Autodesk Fusion 360 part; units mm, degrees
(part 2 of 3)
sketch "Sketch4" plane through (0, 0, 0) normal (0, -1, 0) x (1, 0, 0)
  circle A0 centre (0, 8) radius 4.5
  circle A1 centre (0, 35) radius 5.25
  line L0 (-36.5, 36.5) -> (-36.5, -36.5)
  line L1 (-36.5, -36.5) -> (36.5, -36.5)
  line L2 (36.5, -36.5) -> (36.5, 36.5)
  arc A2 (36.5, 36.5) -> (-36.5, 36.5) centre (0, 36.5) ccw
  line L3 (35, -35) -> (28.75, -35)
  line L4 (28.75, -35) -> (28.75, -30)
  line L5 (28.75, -30) -> (35, -30)
  line L6 (35, -30) -> (35, -35)
  line L7 (28.75, -30) -> (13.75, -30)
  line L8 (13.75, -30) -> (13.75, -20)
  line L9 (13.75, -20) -> (28.75, -20)
  line L10 (28.75, -20) -> (28.75, -30)
  line L11 (13.75, -30) -> (7.5, -30)
  line L12 (7.5, -30) -> (7.5, -35)
  line L13 (7.5, -35) -> (13.75, -35)
  line L14 (13.75, -35) -> (13.75, -30)
  line L15 (7.5, -30) -> (-7.5, -30)
  line L16 (-7.5, -30) -> (-7.5, -20)
  line L17 (-7.5, -20) -> (7.5, -20)
  line L18 (7.5, -20) -> (7.5, -30)
  line L19 (-7.5, -30) -> (-13.75, -30)
  line L20 (-13.75, -30) -> (-13.75, -35)
  line L21 (-13.75, -35) -> (-7.5, -35)
  line L22 (-7.5, -35) -> (-7.5, -30)
  line L23 (-13.75, -30) -> (-28.75, -30)
  line L24 (-28.75, -30) -> (-28.75, -20)
  line L25 (-28.75, -20) -> (-13.75, -20)
  line L26 (-13.75, -20) -> (-13.75, -30)
  line L27 (-28.75, -30) -> (-35, -30)
  line L28 (-35, -30) -> (-35, -35)
  line L29 (-35, -35) -> (-28.75, -35)
  line L30 (-28.75, -35) -> (-28.75, -30)
  line L31 (28.75, -20) -> (35, -20)
  line L32 (35, -20) -> (35, -13.75)
  line L33 (35, -13.75) -> (28.75, -13.75)
  line L34 (28.75, -13.75) -> (28.75, -20)
  line L35 (28.75, -13.75) -> (13.75, -13.75)
  line L36 (13.75, -13.75) -> (13.75, -3.75)
  line L37 (13.75, -3.75) -> (28.75, -3.75)
  line L38 (28.75, -3.75) -> (28.75, -13.75)
  line L39 (13.75, -13.75) -> (7.5, -13.75)
  line L40 (7.5, -13.75) -> (7.5, -20)
  line L41 (7.5, -20) -> (13.75, -20)
  line L42 (13.75, -20) -> (13.75, -13.75)
  line L43 (7.5, -13.75) -> (-7.5, -13.75)
  line L44 (-7.5, -13.75) -> (-7.5, -3.75)
  line L45 (-7.5, -3.75) -> (7.5, -3.75)
  line L46 (7.5, -3.75) -> (7.5, -13.75)
  line L47 (-7.5, -13.75) -> (-13.75, -13.75)
  line L48 (-13.75, -13.75) -> (-13.75, -20)
  line L49 (-13.75, -20) -> (-7.5, -20)
  line L50 (-7.5, -20) -> (-7.5, -13.75)
  line L51 (-13.75, -13.75) -> (-28.75, -13.75)
  line L52 (-28.75, -13.75) -> (-28.75, -3.75)
  line L53 (-28.75, -3.75) -> (-13.75, -3.75)
  line L54 (-13.75, -3.75) -> (-13.75, -13.75)
  point P0 (35, -35)
  point P1 (-35, -35)
  dimension "d22" = 6.25
  dimension "d23" = 5
  dimension "d24" = 15
  dimension "d25" = 10
  dimension "d26" = 6.25
  dimension "d27" = 15
  dimension "d28" = 10
  dimension "d29" = 6.25
  dimension "d30" = 15
  dimension "d31" = 10
  dimension "d32" = 6.25
  dimension "d33" = 15
  dimension "d34" = 10
  dimension "d35" = 15
  dimension "d36" = 10
  dimension "d37" = 15
  dimension "d38" = 10
  constraint horizontal L3
  constraint vertical L4
  constraint horizontal L5
  constraint vertical L6
  constraint coincident P0 L3.start
  constraint horizontal L7
  constraint vertical L8
  constraint horizontal L9
  constraint vertical L10
  constraint horizontal L11
  constraint vertical L12
  constraint horizontal L13
  constraint vertical L14
  constraint horizontal L15
  constraint vertical L16
  constraint horizontal L17
  constraint vertical L18
  constraint horizontal L19
  constraint vertical L20
  constraint horizontal L21
  constraint vertical L22
  constraint horizontal L23
  constraint vertical L24
  constraint horizontal L25
  constraint vertical L26
  constraint horizontal L27
  constraint vertical L28
  constraint horizontal L29
  constraint vertical L30
  constraint coincident P1 L28.end
  constraint horizontal L31
  constraint vertical L32
  constraint horizontal L33
  constraint vertical L34
  constraint horizontal L35
  constraint vertical L36
  constraint horizontal L37
  constraint vertical L38
  constraint horizontal L39
  constraint vertical L40
  constraint horizontal L41
  constraint vertical L42
  constraint horizontal L43
  constraint vertical L44
  constraint horizontal L45
  constraint vertical L46
  constraint horizontal L47
  constraint vertical L48
  constraint horizontal L49
  constraint vertical L50
  constraint horizontal L51
  constraint vertical L52
  constraint horizontal L53
  constraint vertical L54
  measures "d22" distance of P0 L3.end
  measures "d23" distance of P0 L5.end
  measures "d24" distance of L4.end L7.end
  measures "d25" distance of L4.end L9.end
  measures "d26" distance of L7.end L11.end
  measures "d27" distance of L11.end L15.end
  measures "d28" distance of L11.end L17.end
  measures "d29" distance of L15.end L19.end
  measures "d30" distance of L19.end L23.end
  measures "d31" distance of L19.end L25.end
  measures "d32" distance of L9.end L33.end
  measures "d33" distance of L33.end L35.end
  measures "d34" distance of L33.end L37.end
  measures "d35" distance of L39.end L43.end
  measures "d36" distance of L39.end L45.end
  measures "d37" distance of L47.end L51.end
  measures "d38" distance of L47.end L53.end
extrude "Extrude6" cut sketch "Sketch4" against normal blind 3 contours L51 L52 L53 L54 | L7 L8 L9 L10 | L15 L16 L17 L18 | L35 L36 L37 L38 | L43 L44 L45 L46 | L23 L24 L25 L26 bodies 2
sketch "Sketch5" plane through (0, 0, -36.5) normal (0, 0, -1) x (-1, 0, 0)
  line L0 (36.5, 0) -> (-36.5, 0)
  line L1 (-36.5, 0) -> (-36.5, -25)
  line L2 (-36.5, -25) -> (36.5, -25)
  line L3 (36.5, -25) -> (36.5, 0)
  line L4 (36.5, -25) -> (24, -25)
  line L5 (24, -25) -> (24, -16)
  line L6 (24, -16) -> (36.5, -16)
  line L7 (36.5, -16) -> (36.5, -25)
  line L8 (24, -16) -> (11, -16)
  line L9 (11, -16) -> (11, -25)
  line L10 (11, -25) -> (24, -25)
  line L11 (24, -25) -> (24, -16)
  dimension "d41" = 12.5
  dimension "d42" = 9
  dimension "d43" = 13
  constraint horizontal L4
  constraint vertical L5
  constraint horizontal L6
  constraint vertical L7
  constraint coincident L2.end L3.start
  constraint horizontal L8
  constraint vertical L9
  constraint horizontal L10
  constraint vertical L11
  measures "d41" distance of L2.end L4.end
  measures "d42" distance of L2.end L6.end
  measures "d43" distance of L5.end L8.end
extrude "Extrude7" cut sketch "Sketch5" against normal blind 2 contours L2 L5 L8 L9 L10 L11 bodies 1
sketch "Sketch6" plane through (0, 0, 0) normal (0, -1, 0) x (1, 0, 0)
  line L0 (13.75, -13.75) -> (13.75, -3.75)
  line L1 (13.75, -3.75) -> (28.75, -3.75)
  line L2 (28.75, -3.75) -> (28.75, -13.75)
  line L3 (28.75, -13.75) -> (13.75, -13.75)
  line L4 (-28.75, -30) -> (-28.75, -20)
  line L5 (-28.75, -20) -> (-13.75, -20)
  line L6 (-13.75, -20) -> (-13.75, -30)
  line L7 (-13.75, -30) -> (-28.75, -30)
  line L8 (-7.5, -13.75) -> (-7.5, -3.75)
  line L9 (-7.5, -3.75) -> (7.5, -3.75)
  line L10 (7.5, -3.75) -> (7.5, -13.75)
  line L11 (7.5, -13.75) -> (-7.5, -13.75)
  line L12 (13.75, -30) -> (13.75, -20)
  line L13 (13.75, -20) -> (28.75, -20)
  line L14 (28.75, -20) -> (28.75, -30)
  line L15 (28.75, -30) -> (13.75, -30)
  line L16 (-7.5, -30) -> (-7.5, -20)
  line L17 (-7.5, -20) -> (7.5, -20)
  line L18 (7.5, -20) -> (7.5, -30)
  line L19 (7.5, -30) -> (-7.5, -30)
  line L20 (-28.75, -13.75) -> (-28.75, -3.75)
  line L21 (-28.75, -3.75) -> (-13.75, -3.75)
  line L22 (-13.75, -3.75) -> (-13.75, -13.75)
  line L23 (-13.75, -13.75) -> (-28.75, -13.75)
  circle A0 centre (0, 8) radius 4.5
  circle A1 centre (0, 35) radius 5.25
  line L24 (-36.5, 36.5) -> (-36.5, -36.5)
  line L25 (-36.5, -36.5) -> (36.5, -36.5)
  line L26 (36.5, -36.5) -> (36.5, 36.5)
  arc A2 (36.5, 36.5) -> (-36.5, 36.5) centre (0, 36.5) ccw
  circle A3 centre (0, 60) radius 3
  line L27 (31, 7.5) -> (-31, 7.5)
  line L28 (-31, 7.5) -> (-31, -7.5)
  line L29 (-31, -7.5) -> (31, -7.5)
  line L30 (31, -7.5) -> (31, 7.5)
  line L31 (31, 7.5) -> (-31, -7.5) construction
  line L32 (-31, 7.5) -> (31, -7.5) construction
  circle A4 centre (-31, 7.5) radius 1.5
  circle A5 centre (31, 7.5) radius 1.5
  circle A6 centre (-25, 35) radius 2.5
  circle A7 centre (25, 35) radius 2.5
  dimension "d46" = 6
  dimension "d47" = 62
  dimension "d48" = 3
  dimension "d49" = 15
  dimension "d50" = 3
  dimension "d53" = 5
  dimension "d54" = 5
  constraint horizontal L27
  constraint perpendicular L27 L28
  constraint parallel L27 L29
  constraint parallel L28 L30
  constraint coincident L31 origin
  constraint coincident L32 origin
  constraint coincident L27.end L28.start
  constraint coincident L27.start L30.end
  measures "d46" diameter of A3
  measures "d47" distance of L28.end L29.end
  measures "d48" diameter of A4
  measures "d49" distance of L27.start L29.end
  measures "d50" diameter of A5
  measures "d53" diameter of A6
  measures "d54" diameter of A7
extrude "Extrude8" add sketch "Sketch6" along normal blind 20 contours L27 L30 A5 | L27 L30 A5 | L27 L28 A4 | L27 L28 A4 | A3 | A6 | A7 bodies 2

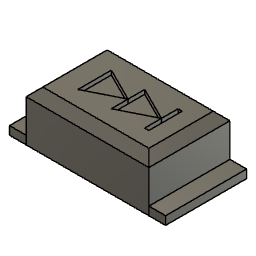
design "klavesa_dopredu_dozadu"
Autodesk Fusion 360 part; units mm, degrees
sketch "Sketch1" plane through (0, 0, 0) normal (0, 1, 0) x (1, 0, 0)
  line L0 (7.35, 4.85) -> (-7.35, 4.85)
  line L1 (-7.35, 4.85) -> (-7.35, -4.85)
  line L2 (-7.35, -4.85) -> (7.35, -4.85)
  line L3 (7.35, -4.85) -> (7.35, 4.85)
  line L4 (7.35, 4.85) -> (-7.35, -4.85) construction
  line L5 (-7.35, 4.85) -> (7.35, -4.85) construction
  line L6 (-7.35, 4.85) -> (-9.35, 4.85)
  line L7 (-9.35, 4.85) -> (-9.35, -4.85)
  line L8 (-9.35, -4.85) -> (-7.35, -4.85)
  line L9 (-7.35, -4.85) -> (-7.35, 4.85)
  line L10 (7.35, 4.85) -> (9.35, 4.85)
  line L11 (9.35, 4.85) -> (9.35, -4.85)
  line L12 (9.35, -4.85) -> (7.35, -4.85)
  line L13 (7.35, -4.85) -> (7.35, 4.85)
  dimension "d1" = 14.7
  dimension "d2" = 9.7
  dimension "d10" = 2
  dimension "d11" = 9.7
  dimension "d12" = 2
  dimension "d13" = 9.7
  constraint horizontal L0
  constraint perpendicular L0 L1
  constraint parallel L0 L2
  constraint parallel L1 L3
  constraint coincident L4 origin
  constraint coincident L5 origin
  constraint horizontal L6
  constraint vertical L7
  constraint horizontal L8
  constraint vertical L9
  constraint horizontal L10
  constraint vertical L11
  constraint horizontal L12
  constraint vertical L13
  measures "d1" distance of L1.end L2.end
  measures "d2" distance of L0.end L1.end
  measures "d10" distance of L0.end L6.end
  measures "d11" distance of L0.end L1.end
  measures "d12" distance of L0.start L10.end
  measures "d13" distance of L0.start L2.end
extrude "Extrude3" add sketch "Sketch1" along normal blind 1 contours L3 L10 L11 L12 L13 | L1 L6 L7 L8 L9 makes body 1 at (8.6833, 0, 1.6167) makes body 2 at (-8.0167, 0, -1.6167)
extrude "Extrude1" add sketch "Sketch1" along normal blind 6 separate body contours L0 L1 L2 L3 L9 L13 makes body 3
chamfer "Chamfer1" distance 1 angle 45 4 edges at (0, 6, 4.85) (7.35, 6, 0) (-7.35, 6, 0) (0, 6, -4.85) measured on face at (-2.45, 6, 1.6167) measured on face at (-2.45, 6, 1.6167) measured on face at (-2.45, 6, 1.6167) measured on face at (-2.45, 6, 1.6167) on bodies 3
sketch "Sketch2" plane through (0, 0, 0) normal (0, -1, 0) x (1, 0, 0)
  line L0 (7.35, -4.85) -> (7.35, 4.85)
  line L1 (7.35, 4.85) -> (-7.35, 4.85)
  line L2 (-7.35, 4.85) -> (-7.35, -4.85)
  line L3 (-7.35, -4.85) -> (7.35, -4.85)
  circle A0 centre (0, 0) radius 1.7
  dimension "d7" = 3.4
  constraint coincident A0.centre origin
  measures "d7" diameter of A0
extrude "Extrude2" cut sketch "Sketch2" against normal blind 4 contours A0 bodies 3
sketch "Sketch4" plane through (0, 6, 0) normal (0, 1, 0) x (-1, 0, 0)
  line L0 (-6.35, -3.85) -> (6.35, -3.85)
  line L1 (6.35, -3.85) -> (6.35, 3.85)
  line L2 (6.35, 3.85) -> (-6.35, 3.85)
  line L3 (-6.35, 3.85) -> (-6.35, -3.85)
  line L4 (-4, -2) -> (4, -2)
  line L5 (4, -2) -> (4, 2)
  line L6 (4, 2) -> (-4, 2)
  line L7 (-4, 2) -> (-4, -2)
  line L8 (-4, -2) -> (4, 2) construction
  line L9 (4, -2) -> (-4, 2) construction
  line L10 (4, -2) -> (0, -2)
  line L11 (0, -2) -> (0, 2)
  line L12 (0, 2) -> (4, 2)
  line L13 (4, 2) -> (4, -2)
  line L14 (4, -2) -> (0, 0)
  line L15 (4, 2) -> (0, 0)
  line L16 (0, -2) -> (-4, 0)
  line L17 (0, 2) -> (-4, 0)
  line L18 (-4, -2) -> (-4.5, -2)
  line L19 (-4.5, -2) -> (-4.5, 2)
  line L20 (-4.5, 2) -> (-4, 2)
  line L21 (-4, 2) -> (-4, -2)
  dimension "d25" = 8
  dimension "d26" = 4
  dimension "d27" = 0.5
  constraint horizontal L4
  constraint perpendicular L4 L5
  constraint parallel L4 L6
  constraint parallel L5 L7
  constraint coincident L8 L14.end
  constraint coincident L9 L14.end
  constraint coincident L14.end L15.end
  constraint horizontal L10
  constraint vertical L11
  constraint horizontal L12
  constraint vertical L13
  constraint midpoint L6 L11.end
  constraint midpoint L7 L16.end
  constraint horizontal L18
  constraint vertical L19
  constraint horizontal L20
  constraint vertical L21
  measures "d25" distance of L5.end L6.end
  measures "d26" distance of L4.end L5.end
  measures "d27" distance of L4.start L18.end
extrude "Extrude5" cut sketch "Sketch4" against normal blind 0.5 contours L7 L18 L19 L20 L21 | L11 L16 L17 | L5 L13 L14 L15 bodies 3

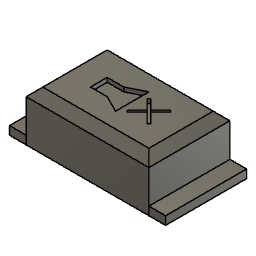
design "klavesa_mute"
Autodesk Fusion 360 part; units mm, degrees
sketch "Sketch1" plane through (0, 0, 0) normal (0, 1, 0) x (1, 0, 0)
  line L0 (7.35, 4.85) -> (-7.35, 4.85)
  line L1 (-7.35, 4.85) -> (-7.35, -4.85)
  line L2 (-7.35, -4.85) -> (7.35, -4.85)
  line L3 (7.35, -4.85) -> (7.35, 4.85)
  line L4 (7.35, 4.85) -> (-7.35, -4.85) construction
  line L5 (-7.35, 4.85) -> (7.35, -4.85) construction
  line L6 (-7.35, 4.85) -> (-9.35, 4.85)
  line L7 (-9.35, 4.85) -> (-9.35, -4.85)
  line L8 (-9.35, -4.85) -> (-7.35, -4.85)
  line L9 (-7.35, -4.85) -> (-7.35, 4.85)
  line L10 (7.35, 4.85) -> (9.35, 4.85)
  line L11 (9.35, 4.85) -> (9.35, -4.85)
  line L12 (9.35, -4.85) -> (7.35, -4.85)
  line L13 (7.35, -4.85) -> (7.35, 4.85)
  dimension "d1" = 14.7
  dimension "d2" = 9.7
  dimension "d10" = 2
  dimension "d11" = 9.7
  dimension "d12" = 2
  dimension "d13" = 9.7
  constraint horizontal L0
  constraint perpendicular L0 L1
  constraint parallel L0 L2
  constraint parallel L1 L3
  constraint coincident L4 origin
  constraint coincident L5 origin
  constraint horizontal L6
  constraint vertical L7
  constraint horizontal L8
  constraint vertical L9
  constraint horizontal L10
  constraint vertical L11
  constraint horizontal L12
  constraint vertical L13
  measures "d1" distance of L1.end L2.end
  measures "d2" distance of L0.end L1.end
  measures "d10" distance of L0.end L6.end
  measures "d11" distance of L0.end L1.end
  measures "d12" distance of L0.start L10.end
  measures "d13" distance of L0.start L2.end
extrude "Extrude3" add sketch "Sketch1" along normal blind 1 contours L3 L10 L11 L12 L13 | L1 L6 L7 L8 L9 makes body 1 at (8.6833, 0, 1.6167) makes body 2 at (-8.0167, 0, -1.6167)
extrude "Extrude1" add sketch "Sketch1" along normal blind 6 separate body contours L0 L1 L2 L3 L9 L13 makes body 3
chamfer "Chamfer1" distance 1 angle 45 4 edges at (0, 6, 4.85) (7.35, 6, 0) (-7.35, 6, 0) (0, 6, -4.85) measured on face at (-2.45, 6, 1.6167) measured on face at (-2.45, 6, 1.6167) measured on face at (-2.45, 6, 1.6167) measured on face at (-2.45, 6, 1.6167) on bodies 3
sketch "Sketch2" plane through (0, 0, 0) normal (0, -1, 0) x (1, 0, 0)
  line L0 (7.35, -4.85) -> (7.35, 4.85)
  line L1 (7.35, 4.85) -> (-7.35, 4.85)
  line L2 (-7.35, 4.85) -> (-7.35, -4.85)
  line L3 (-7.35, -4.85) -> (7.35, -4.85)
  circle A0 centre (0, 0) radius 1.7
  dimension "d7" = 3.4
  constraint coincident A0.centre origin
  measures "d7" diameter of A0
extrude "Extrude2" cut sketch "Sketch2" against normal blind 4 contours A0 bodies 3
sketch "Sketch3" plane through (0, 6, 0) normal (0, 1, 0) x (-1, 0, 0)
  line L0 (-6.35, -3.85) -> (6.35, -3.85)
  line L1 (6.35, -3.85) -> (6.35, 3.85)
  line L2 (6.35, 3.85) -> (-6.35, 3.85)
  line L3 (-6.35, 3.85) -> (-6.35, -3.85)
  line L4 (-4, -2.5) -> (4, -2.5)
  line L5 (4, -2.5) -> (4, 2.5)
  line L6 (4, 2.5) -> (-4, 2.5)
  line L7 (-4, 2.5) -> (-4, -2.5)
  line L8 (-4, -2.5) -> (4, 2.5) construction
  line L9 (4, -2.5) -> (-4, 2.5) construction
  line L10 (1.5, -1) -> (3.5, -1)
  line L11 (3.5, -1) -> (3.5, 1)
  line L12 (3.5, 1) -> (1.5, 1)
  line L13 (1.5, 1) -> (1.5, -1)
  line L14 (1.5, -1) -> (3.5, 1) construction
  line L15 (3.5, -1) -> (1.5, 1) construction
  line L16 (-0.5, -2) -> (1.5, -2)
  line L17 (1.5, -2) -> (1.5, 2)
  line L18 (1.5, 2) -> (-0.5, 2)
  line L19 (-0.5, 2) -> (-0.5, -2)
  line L20 (-0.5, -2) -> (1.5, 2) construction
  line L21 (1.5, -2) -> (-0.5, 2) construction
  line L22 (1.5, -1) -> (-0.5, -2)
  line L23 (1.5, 1) -> (-0.5, 2)
  line L24 (-1, 1.5) -> (-4, 1.5)
  line L25 (-4, 1.5) -> (-4, -1.5)
  line L26 (-4, -1.5) -> (-1, -1.5)
  line L27 (-1, -1.5) -> (-1, 1.5)
  line L28 (-1, 1.5) -> (-4, -1.5) construction
  line L29 (-4, 1.5) -> (-1, -1.5) construction
  line L30 (-2.5, 0) -> (-1.2, -1.3)
  line L31 (-1.2, -1.3) -> (-1.3061, -1.4061)
  line L32 (-1.3061, -1.4061) -> (-2.6061, -0.1061)
  line L33 (-2.6061, -0.1061) -> (-2.5, 0)
  line L34 (-2.5, 0) -> (-1.2, -1.3)
  line L35 (-1.2, -1.3) -> (-1.0939, -1.1939)
  line L36 (-1.0939, -1.1939) -> (-2.3939, 0.1061)
  line L37 (-2.3939, 0.1061) -> (-2.5, 0)
  line L38 (-2.5, 0) -> (-3.8, 1.3)
  line L39 (-3.8, 1.3) -> (-3.9061, 1.1939)
  line L40 (-3.9061, 1.1939) -> (-2.6061, -0.1061)
  line L41 (-2.6061, -0.1061) -> (-2.5, 0)
  line L42 (-2.5, 0) -> (-3.8, 1.3)
  line L43 (-3.8, 1.3) -> (-3.6939, 1.4061)
  line L44 (-3.6939, 1.4061) -> (-2.3939, 0.1061)
  line L45 (-2.3939, 0.1061) -> (-2.5, 0)
  line L46 (-2.5, 0) -> (-1.2, 1.3)
  line L47 (-1.2, 1.3) -> (-1.0939, 1.1939)
  line L48 (-1.0939, 1.1939) -> (-2.3939, -0.1061)
  line L49 (-2.3939, -0.1061) -> (-2.5, 0)
  line L50 (-2.5, 0) -> (-1.2, 1.3)
  line L51 (-1.2, 1.3) -> (-1.3061, 1.4061)
  line L52 (-1.3061, 1.4061) -> (-2.6061, 0.1061)
  line L53 (-2.6061, 0.1061) -> (-2.5, 0)
  line L54 (-2.5, 0) -> (-3.8, -1.3)
  line L55 (-3.8, -1.3) -> (-3.6939, -1.4061)
  line L56 (-3.6939, -1.4061) -> (-2.3939, -0.1061)
  line L57 (-2.3939, -0.1061) -> (-2.5, 0)
  line L58 (-2.5, 0) -> (-3.8, -1.3)
  line L59 (-3.8, -1.3) -> (-3.9061, -1.1939)
  line L60 (-3.9061, -1.1939) -> (-2.6061, 0.1061)
  line L61 (-2.6061, 0.1061) -> (-2.5, 0)
  point P0 (2, 0)
  point P1 (2.5, 0)
  point P2 (0.5, 0)
  point P3 (-2.5, 0)
  dimension "d17" = 2
  dimension "d18" = 2
  dimension "d19" = 2
  dimension "d20" = 4
  dimension "d21" = 3
  dimension "d22" = 3
  dimension "d25" = 0.15
  dimension "d26" = 0.15
  dimension "d27" = 0.15
  dimension "d28" = 0.15
  dimension "d29" = 0.15
  dimension "d30" = 0.15
  dimension "d31" = 0.15
  dimension "d32" = 0.15
  constraint horizontal L4
  constraint perpendicular L4 L5
  constraint parallel L4 L6
  constraint parallel L5 L7
  constraint coincident L8 origin
  constraint coincident L9 origin
  constraint horizontal L10
  constraint perpendicular L10 L11
  constraint parallel L10 L12
  constraint parallel L11 L13
  constraint coincident L14 P1
  constraint coincident L15 P1
  constraint horizontal L16
  constraint perpendicular L16 L17
  constraint parallel L16 L18
  constraint parallel L17 L19
  constraint coincident L20 P2
  constraint coincident L21 P2
  constraint horizontal L24
  constraint perpendicular L24 L25
  constraint parallel L24 L26
  constraint parallel L25 L27
  constraint coincident L28 P3
  constraint coincident L29 P3
  constraint perpendicular L30 L31
  constraint parallel L30 L32
  constraint parallel L31 L33
  constraint coincident L29 L30.end
  constraint perpendicular L28 L30
  constraint coincident P3 L30.start
  constraint perpendicular L34 L35
  constraint parallel L34 L36
  constraint parallel L35 L37
  constraint perpendicular L31 L34
  constraint perpendicular L38 L39
  constraint parallel L38 L40
  constraint parallel L39 L41
  constraint coincident L29 L38.end
  constraint perpendicular L42 L43
  constraint parallel L42 L44
  constraint parallel L43 L45
  constraint perpendicular L46 L47
  constraint parallel L46 L48
  constraint parallel L47 L49
  constraint coincident L28 L46.end
  constraint perpendicular L30 L46
  constraint perpendicular L50 L51
  constraint parallel L50 L52
  constraint parallel L51 L53
  constraint perpendicular L54 L55
  constraint parallel L54 L56
  constraint parallel L55 L57
  constraint coincident L28 L54.end
  constraint parallel L28 L54
  constraint perpendicular L58 L59
  constraint parallel L58 L60
  constraint parallel L59 L61
  measures "d17" distance of L11.end L12.end
  measures "d18" distance of L10.end L11.end
  measures "d19" distance of L17.end L18.end
  measures "d20" distance of L16.end L17.end
  measures "d21" distance of L25.end L26.end
  measures "d22" distance of L24.end L25.end
  measures "d25" distance of P3 L32.end
  measures "d26" distance of P3 L36.end
  measures "d27" distance of P3 L32.end
  measures "d28" distance of P3 L36.end
  measures "d29" distance of P3 L48.end
  measures "d30" distance of P3 L52.end
  measures "d31" distance of P3 L48.end
  measures "d32" distance of P3 L52.end
extrude "Extrude4" cut sketch "Sketch3" against normal blind 0.5 contours L10 L11 L12 L13 L17 | L13 L17 L19 L22 L23 | L30 L34 L36 L37 L45 L46 L48 L49 L50 L57 | L30 L32 L33 L34 L41 L49 L54 L56 L57 L58 | L37 L38 L42 L44 L45 L46 L50 L52 L53 L61 | L33 L38 L40 L41 L42 L53 L54 L58 L60 L61 | L30 L34 L35 L36 L48 | L30 L31 L32 L34 L56 | L40 L54 L58 L59 L60 | L32 L54 L55 L56 L58 | L36 L46 L47 L48 L50 | L44 L46 L50 L51 L52 | L38 L39 L40 L42 L60 | L38 L42 L43 L44 L52 bodies 3

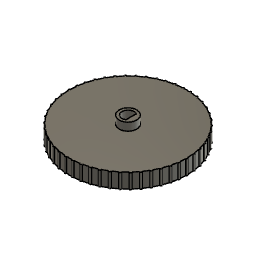
design "big_circle"
Autodesk Fusion 360 part; units mm, degrees
sketch "Sketch1" plane through (0, 0, 0) normal (0, 1, 0) x (1, 0, 0)
  circle A0 centre (0, 0) radius 30
  dimension "d1" = 60
  constraint coincident A0.centre origin
  measures "d1" diameter of A0
extrude "Extrude1" add sketch "Sketch1" along normal blind 7.5
sketch "Sketch2" plane through (0, 7.5, 0) normal (0, 1, 0) x (-1, 0, 0)
  circle A0 centre (0, 0) radius 30
  circle A1 centre (0, 0) radius 4.5
  dimension "d4" = 9
  constraint concentric A0 A1
  measures "d4" diameter of A1
extrude "Extrude2" add sketch "Sketch2" along normal blind 4 contours A1
sketch "Sketch3" plane through (0, 11.5, 0) normal (0, 1, 0) x (-1, 0, 0)
  circle A0 centre (0, 0) radius 4.5
  circle A1 centre (0, 0) radius 3.075
  line L0 (3.075, 0) -> (-1.575, 0)
  line L1 (-1.575, 0) -> (-1.575, -0.2)
  line L2 (-1.575, -0.2) -> (3.075, -0.2)
  line L3 (3.075, -0.2) -> (3.075, 0)
  line L4 (-1.575, -0.2) -> (-3.025, -0.2)
  line L5 (-3.025, -0.2) -> (-3.025, -2.7)
  line L6 (-3.025, -2.7) -> (-1.575, -2.7)
  line L7 (-1.575, -2.7) -> (-1.575, -0.2)
  line L8 (-1.575, -0.2) -> (-3.025, -0.2)
  line L9 (-3.025, -0.2) -> (-3.025, 2.8)
  line L10 (-3.025, 2.8) -> (-1.575, 2.8)
  line L11 (-1.575, 2.8) -> (-1.575, -0.2)
  dimension "d7" = 6.15
  dimension "d8" = 4.65
  constraint concentric A0 A1
  constraint horizontal L0
  constraint vertical L1
  constraint horizontal L2
  constraint vertical L3
  constraint coincident A1 L0.start
  constraint horizontal L4
  constraint vertical L5
  constraint horizontal L6
  constraint vertical L7
  constraint horizontal L8
  constraint vertical L9
  constraint horizontal L10
  constraint vertical L11
  measures "d7" diameter of A1
  measures "d8" distance of L0.start L0.end
extrude "Extrude3" cut sketch "Sketch3" against normal blind 9 contours A1 L0 L11 | A1 L0 L1 L2 L11 | A1 L2 L7
sketch "Sketch6" plane through (0, 0, 0) normal (0, -1, 0) x (1, 0, 0)
  circle A0 centre (0, 0) radius 30
  circle A1 centre (-30, 0) radius 0.5
  circle A2 centre (-29.7634, -3.76) radius 0.5
  circle A3 centre (-29.0575, -7.4607) radius 0.5
  circle A4 centre (-27.8933, -11.0437) radius 0.5
  circle A5 centre (-26.2892, -14.4526) radius 0.5
  circle A6 centre (-24.2705, -17.6336) radius 0.5
  circle A7 centre (-21.8691, -20.5364) radius 0.5
  circle A8 centre (-19.1227, -23.1154) radius 0.5
  circle A9 centre (-16.0748, -25.3298) radius 0.5
  circle A10 centre (-12.7734, -27.1448) radius 0.5
  circle A11 centre (-9.2705, -28.5317) radius 0.5
  circle A12 centre (-5.6214, -29.4686) radius 0.5
  circle A13 centre (-1.8837, -29.9408) radius 0.5
  circle A14 centre (1.8837, -29.9408) radius 0.5
  circle A15 centre (5.6214, -29.4686) radius 0.5
  circle A16 centre (9.2705, -28.5317) radius 0.5
  circle A17 centre (12.7734, -27.1448) radius 0.5
  circle A18 centre (16.0748, -25.3298) radius 0.5
  circle A19 centre (19.1227, -23.1154) radius 0.5
  circle A20 centre (21.8691, -20.5364) radius 0.5
  circle A21 centre (24.2705, -17.6336) radius 0.5
  circle A22 centre (26.2892, -14.4526) radius 0.5
  circle A23 centre (27.8933, -11.0437) radius 0.5
  circle A24 centre (29.0575, -7.4607) radius 0.5
  circle A25 centre (29.7634, -3.76) radius 0.5
  circle A26 centre (30, 0) radius 0.5
  circle A27 centre (29.7634, 3.76) radius 0.5
  circle A28 centre (29.0575, 7.4607) radius 0.5
  circle A29 centre (27.8933, 11.0437) radius 0.5
  circle A30 centre (26.2892, 14.4526) radius 0.5
  circle A31 centre (24.2705, 17.6336) radius 0.5
  circle A32 centre (21.8691, 20.5364) radius 0.5
  circle A33 centre (19.1227, 23.1154) radius 0.5
  circle A34 centre (16.0748, 25.3298) radius 0.5
  circle A35 centre (12.7734, 27.1448) radius 0.5
  circle A36 centre (9.2705, 28.5317) radius 0.5
  circle A37 centre (5.6214, 29.4686) radius 0.5
  circle A38 centre (1.8837, 29.9408) radius 0.5
  circle A39 centre (-1.8837, 29.9408) radius 0.5
  circle A40 centre (-5.6214, 29.4686) radius 0.5
  circle A41 centre (-9.2705, 28.5317) radius 0.5
  circle A42 centre (-12.7734, 27.1448) radius 0.5
  circle A43 centre (-16.0748, 25.3298) radius 0.5
  circle A44 centre (-19.1227, 23.1154) radius 0.5
  circle A45 centre (-21.8691, 20.5364) radius 0.5
  circle A46 centre (-24.2705, 17.6336) radius 0.5
  circle A47 centre (-26.2892, 14.4526) radius 0.5
  circle A48 centre (-27.8933, 11.0437) radius 0.5
  circle A49 centre (-29.0575, 7.4607) radius 0.5
  circle A50 centre (-29.7634, 3.76) radius 0.5
  dimension "d11" = 1
  dimension "d15" = 360
  constraint coincident A0 A1.centre
  measures "d11" diameter of A1
extrude "Extrude4" add sketch "Sketch6" against normal blind 7.5 contours A0 A26 | A0 A27 | A0 A25 | A0 A28 | A0 A24 | A0 A29 | A0 A23 | A0 A30 | A0 A22 | A0 A31 | A0 A21 | A0 A32 | A0 A20 | A0 A33 | A0 A19 | A0 A34 | A0 A18 | A0 A35 | A0 A17 | A0 A36 | A0 A16 | A0 A37 | A0 A15 | A0 A38 | A0 A14 | A0 A39 | A0 A13 | A0 A40 | A0 A12 | A0 A41 | A0 A11 | A0 A42 | A0 A10 | A0 A43 | A0 A9 | A0 A44 | A0 A8 | A0 A45 | A0 A7 | A0 A46 | A0 A6 | A0 A47 | A0 A5 | A0 A48 | A0 A4 | A0 A49 | A0 A3 | A0 A50 | A0 A2 | A0 A1 picked at (30.1597, -0.1028) picked at (29.9281, 3.7836) picked at (29.9281, -3.7836) picked at (29.2173, 7.5069) picked at (29.2173, -7.5069) picked at (28.0452, 11.1115) picked at (28.0452, -11.1115) picked at (26.4393, 14.5244) picked at (26.4393, -14.5244) picked at (24.4089, 17.7259) picked at (24.4089, -17.7259) picked at (21.9931, 20.6472) picked at (21.9931, -20.6472) picked at (19.2303, 23.2423) picked at (19.2303, -23.2423) picked at (16.164, 25.4703) picked at (16.164, -25.4703) picked at (12.8427, 27.296) picked at (12.8427, -27.296) picked at (9.3317, 28.6864) picked at (9.3317, -28.6864) picked at (5.6607, 29.6303) picked at (5.6607, -29.6303) picked at (1.9005, 30.1063) picked at (1.9005, -30.1063) picked at (-1.8942, 30.1068) picked at (-1.8942, -30.1068) picked at (-5.6526, 29.632) picked at (-5.6526, -29.632) picked at (-9.3219, 28.6899) picked at (-9.3219, -28.6899) picked at (-12.8442, 27.2953) picked at (-12.8442, -27.2953) picked at (-16.1639, 25.4703) picked at (-16.1639, -25.4703) picked at (-19.2288, 23.2436) picked at (-19.2288, -23.2436) picked at (-21.9903, 20.6503) picked at (-21.9903, -20.6503) picked at (-24.4051, 17.7313) picked at (-24.4051, -17.7313) picked at (-26.435, 14.5328) picked at (-26.435, -14.5328) picked at (-28.048, 11.105) picked at (-28.048, -11.105) picked at (-29.2186, 7.5021) picked at (-29.2186, -7.5021) picked at (-29.9285, 3.7808) picked at (-29.9285, -3.7808) picked at (-30.1664, 0)
sketch "Sketch9" plane through (0, 0, 0) normal (0, -1, 0) x (1, 0, 0)
  arc A0 (-24.561, 17.2266) -> (-26.0447, 14.8887) centre (0, 0) ccw
  arc A1 (-26.0447, 14.8887) -> (-26.5264, 14.0125) centre (-26.2892, 14.4526) ccw
  arc A2 (-26.5264, 14.0125) -> (-27.7054, 11.5071) centre (0, 0) ccw
  arc A3 (-27.7054, 11.5071) -> (-28.0735, 10.5773) centre (-27.8933, 11.0437) ccw
  arc A4 (-28.0735, 10.5773) -> (-28.9291, 7.9439) centre (0, 0) ccw
  arc A5 (-28.9291, 7.9439) -> (-29.1778, 6.9754) centre (-29.0575, 7.4607) ccw
  arc A6 (-29.1778, 6.9754) -> (-29.6966, 4.2555) centre (0, 0) ccw
  arc A7 (-29.6966, 4.2555) -> (-29.822, 3.2634) centre (-29.7634, 3.76) ccw
  arc A8 (-29.822, 3.2634) -> (-29.9958, 0.5) centre (0, 0) ccw
  arc A9 (-29.9958, 0.5) -> (-29.9958, -0.5) centre (-30, 0) ccw
  arc A10 (-29.9958, -0.5) -> (-29.822, -3.2634) centre (0, 0) ccw
  arc A11 (-29.822, -3.2634) -> (-29.6966, -4.2555) centre (-29.7634, -3.76) ccw
  arc A12 (-29.6966, -4.2555) -> (-29.1778, -6.9754) centre (0, 0) ccw
  arc A13 (-29.1778, -6.9754) -> (-28.9291, -7.9439) centre (-29.0575, -7.4607) ccw
  arc A14 (-28.9291, -7.9439) -> (-28.0735, -10.5773) centre (0, 0) ccw
  arc A15 (-28.0735, -10.5773) -> (-27.7054, -11.5071) centre (-27.8933, -11.0437) ccw
  arc A16 (-27.7054, -11.5071) -> (-26.5264, -14.0125) centre (0, 0) ccw
  arc A17 (-26.5264, -14.0125) -> (-26.0447, -14.8887) centre (-26.2892, -14.4526) ccw
  arc A18 (-26.0447, -14.8887) -> (-24.561, -17.2266) centre (0, 0) ccw
  arc A19 (-24.561, -17.2266) -> (-23.9733, -18.0356) centre (-24.2705, -17.6336) ccw
  arc A20 (-23.9733, -18.0356) -> (-22.2083, -20.1691) centre (0, 0) ccw
  arc A21 (-22.2083, -20.1691) -> (-21.5238, -20.898) centre (-21.8691, -20.5364) ccw
  arc A22 (-21.5238, -20.898) -> (-19.5053, -22.7935) centre (0, 0) ccw
  arc A23 (-19.5053, -22.7935) -> (-18.7348, -23.4309) centre (-19.1227, -23.1154) ccw
  arc A24 (-18.7348, -23.4309) -> (-16.4947, -25.0584) centre (0, 0) ccw
  arc A25 (-16.4947, -25.0584) -> (-15.6504, -25.5942) centre (-16.0748, -25.3298) ccw
  arc A26 (-15.6504, -25.5942) -> (-13.224, -26.9282) centre (0, 0) ccw
  arc A27 (-13.224, -26.9282) -> (-12.3192, -27.3539) centre (-12.7734, -27.1448) ccw
  arc A28 (-12.3192, -27.3539) -> (-9.7447, -28.3732) centre (0, 0) ccw
  arc A29 (-9.7447, -28.3732) -> (-8.7937, -28.6822) centre (-9.2705, -28.5317) ccw
  arc A30 (-8.7937, -28.6822) -> (-6.1118, -29.3708) centre (0, 0) ccw
  arc A31 (-6.1118, -29.3708) -> (-5.1295, -29.5582) centre (-5.6214, -29.4686) ccw
  arc A32 (-5.1295, -29.5582) -> (-2.3824, -29.9052) centre (0, 0) ccw
  arc A33 (-2.3824, -29.9052) -> (-1.3845, -29.968) centre (-1.8837, -29.9408) ccw
  arc A34 (-1.3845, -29.968) -> (1.3845, -29.968) centre (0, 0) ccw
  arc A35 (1.3845, -29.968) -> (2.3824, -29.9052) centre (1.8837, -29.9408) ccw
  arc A36 (2.3824, -29.9052) -> (5.1295, -29.5582) centre (0, 0) ccw
  arc A37 (5.1295, -29.5582) -> (6.1118, -29.3708) centre (5.6214, -29.4686) ccw
  arc A38 (6.1118, -29.3708) -> (8.7937, -28.6822) centre (0, 0) ccw
  arc A39 (8.7937, -28.6822) -> (9.7447, -28.3732) centre (9.2705, -28.5317) ccw
  arc A40 (9.7447, -28.3732) -> (12.3192, -27.3539) centre (0, 0) ccw
  arc A41 (12.3192, -27.3539) -> (13.224, -26.9282) centre (12.7734, -27.1448) ccw
  arc A42 (13.224, -26.9282) -> (15.6504, -25.5942) centre (0, 0) ccw
  arc A43 (15.6504, -25.5942) -> (16.4947, -25.0584) centre (16.0748, -25.3298) ccw
  arc A44 (16.4947, -25.0584) -> (18.7348, -23.4309) centre (0, 0) ccw
  arc A45 (18.7348, -23.4309) -> (19.5053, -22.7935) centre (19.1227, -23.1154) ccw
  arc A46 (19.5053, -22.7935) -> (21.5238, -20.898) centre (0, 0) ccw
  arc A47 (21.5238, -20.898) -> (22.2083, -20.1691) centre (21.8691, -20.5364) ccw
  arc A48 (22.2083, -20.1691) -> (23.9733, -18.0356) centre (0, 0) ccw
  arc A49 (23.9733, -18.0356) -> (24.561, -17.2266) centre (24.2705, -17.6336) ccw
  arc A50 (24.561, -17.2266) -> (26.0447, -14.8887) centre (0, 0) ccw
  arc A51 (26.0447, -14.8887) -> (26.5264, -14.0125) centre (26.2892, -14.4526) ccw
  arc A52 (26.5264, -14.0125) -> (27.7054, -11.5071) centre (0, 0) ccw
  arc A53 (27.7054, -11.5071) -> (28.0735, -10.5773) centre (27.8933, -11.0437) ccw
  arc A54 (28.0735, -10.5773) -> (28.9291, -7.9439) centre (0, 0) ccw
  arc A55 (28.9291, -7.9439) -> (29.1778, -6.9754) centre (29.0575, -7.4607) ccw
  arc A56 (29.1778, -6.9754) -> (29.6966, -4.2555) centre (0, 0) ccw
  arc A57 (29.6966, -4.2555) -> (29.822, -3.2634) centre (29.7634, -3.76) ccw
  arc A58 (29.822, -3.2634) -> (29.9958, -0.5) centre (0, 0) ccw
  arc A59 (29.9958, -0.5) -> (29.9958, 0.5) centre (30, 0) ccw
  arc A60 (29.9958, 0.5) -> (29.822, 3.2634) centre (0, 0) ccw
  arc A61 (29.822, 3.2634) -> (29.6966, 4.2555) centre (29.7634, 3.76) ccw
  arc A62 (29.6966, 4.2555) -> (29.1778, 6.9754) centre (0, 0) ccw
  arc A63 (29.1778, 6.9754) -> (28.9291, 7.9439) centre (29.0575, 7.4607) ccw
  arc A64 (28.9291, 7.9439) -> (28.0735, 10.5773) centre (0, 0) ccw
  arc A65 (28.0735, 10.5773) -> (27.7054, 11.5071) centre (27.8933, 11.0437) ccw
  arc A66 (27.7054, 11.5071) -> (26.5264, 14.0125) centre (0, 0) ccw
  arc A67 (26.5264, 14.0125) -> (26.0447, 14.8887) centre (26.2892, 14.4526) ccw
  arc A68 (26.0447, 14.8887) -> (24.561, 17.2266) centre (0, 0) ccw
  arc A69 (24.561, 17.2266) -> (23.9733, 18.0356) centre (24.2705, 17.6336) ccw
  arc A70 (23.9733, 18.0356) -> (22.2083, 20.1691) centre (0, 0) ccw
  arc A71 (22.2083, 20.1691) -> (21.5238, 20.898) centre (21.8691, 20.5364) ccw
  arc A72 (21.5238, 20.898) -> (19.5053, 22.7935) centre (0, 0) ccw
  arc A73 (19.5053, 22.7935) -> (18.7348, 23.4309) centre (19.1227, 23.1154) ccw
  arc A74 (18.7348, 23.4309) -> (16.4947, 25.0584) centre (0, 0) ccw
  arc A75 (16.4947, 25.0584) -> (15.6504, 25.5942) centre (16.0748, 25.3298) ccw
  arc A76 (15.6504, 25.5942) -> (13.224, 26.9282) centre (0, 0) ccw
  arc A77 (13.224, 26.9282) -> (12.3192, 27.3539) centre (12.7734, 27.1448) ccw
  arc A78 (12.3192, 27.3539) -> (9.7447, 28.3732) centre (0, 0) ccw
  arc A79 (9.7447, 28.3732) -> (8.7937, 28.6822) centre (9.2705, 28.5317) ccw
  arc A80 (8.7937, 28.6822) -> (6.1118, 29.3708) centre (0, 0) ccw
  arc A81 (6.1118, 29.3708) -> (5.1295, 29.5582) centre (5.6214, 29.4686) ccw
  arc A82 (5.1295, 29.5582) -> (2.3824, 29.9052) centre (0, 0) ccw
  arc A83 (2.3824, 29.9052) -> (1.3845, 29.968) centre (1.8837, 29.9408) ccw
  arc A84 (1.3845, 29.968) -> (-1.3845, 29.968) centre (0, 0) ccw
  arc A85 (-1.3845, 29.968) -> (-2.3824, 29.9052) centre (-1.8837, 29.9408) ccw
  arc A86 (-2.3824, 29.9052) -> (-5.1295, 29.5582) centre (0, 0) ccw
  arc A87 (-5.1295, 29.5582) -> (-6.1118, 29.3708) centre (-5.6214, 29.4686) ccw
  arc A88 (-6.1118, 29.3708) -> (-8.7937, 28.6822) centre (0, 0) ccw
  arc A89 (-8.7937, 28.6822) -> (-9.7447, 28.3732) centre (-9.2705, 28.5317) ccw
  arc A90 (-9.7447, 28.3732) -> (-12.3192, 27.3539) centre (0, 0) ccw
  arc A91 (-12.3192, 27.3539) -> (-13.224, 26.9282) centre (-12.7734, 27.1448) ccw
  arc A92 (-13.224, 26.9282) -> (-15.6504, 25.5942) centre (0, 0) ccw
  arc A93 (-15.6504, 25.5942) -> (-16.4947, 25.0584) centre (-16.0748, 25.3298) ccw
  arc A94 (-16.4947, 25.0584) -> (-18.7348, 23.4309) centre (0, 0) ccw
  arc A95 (-18.7348, 23.4309) -> (-19.5053, 22.7935) centre (-19.1227, 23.1154) ccw
  arc A96 (-19.5053, 22.7935) -> (-21.5238, 20.898) centre (0, 0) ccw
  arc A97 (-21.5238, 20.898) -> (-22.2083, 20.1691) centre (-21.8691, 20.5364) ccw
  arc A98 (-22.2083, 20.1691) -> (-23.9733, 18.0356) centre (0, 0) ccw
  arc A99 (-23.9733, 18.0356) -> (-24.561, 17.2266) centre (-24.2705, 17.6336) ccw
  line L0 (22.5, 15) -> (-22.5, 15)
  line L1 (-22.5, 15) -> (-22.5, -15)
  line L2 (-22.5, -15) -> (22.5, -15)
  line L3 (22.5, -15) -> (22.5, 15)
  line L4 (22.5, 15) -> (-22.5, -15) construction
  line L5 (-22.5, 15) -> (22.5, -15) construction
  line L6 (-22.5, 15) -> (-10, 15)
  line L7 (-10, 15) -> (-10, -15)
  line L8 (-10, -15) -> (-22.5, -15)
  line L9 (-22.5, -15) -> (-22.5, 15)
  line L10 (0, 10) -> (-20, 10)
  line L11 (-20, 10) -> (-20, -10)
  line L12 (-20, -10) -> (0, -10)
  line L13 (0, -10) -> (0, 10)
  line L14 (0, 10) -> (-20, -10) construction
  line L15 (-20, 10) -> (0, -10) construction
  line L16 (-20, 10) -> (0, 0)
  line L17 (-20, -10) -> (0, 0)
  line L18 (22.5, 15) -> (10, 15)
  line L19 (10, 15) -> (10, -15)
  line L20 (10, -15) -> (22.5, -15)
  line L21 (22.5, -15) -> (22.5, 15)
  line L22 (20, 10) -> (0, 10)
  line L23 (0, 10) -> (0, -10)
  line L24 (0, -10) -> (20, -10)
  line L25 (20, -10) -> (20, 10)
  line L26 (20, 10) -> (0, -10) construction
  line L27 (0, 10) -> (20, -10) construction
  line L28 (15, 1) -> (5, 1)
  line L29 (5, 1) -> (5, -1)
  line L30 (5, -1) -> (15, -1)
  line L31 (15, -1) -> (15, 1)
  line L32 (15, 1) -> (5, -1) construction
  line L33 (5, 1) -> (15, -1) construction
  line L34 (17.5, 10) -> (12.5, 10)
  line L35 (12.5, 10) -> (12.5, -10)
  line L36 (12.5, -10) -> (17.5, -10)
  line L37 (17.5, -10) -> (17.5, 10)
  line L38 (17.5, 10) -> (12.5, -10) construction
  line L39 (12.5, 10) -> (17.5, -10) construction
  line L40 (7.5, 10) -> (2.5, 10)
  line L41 (2.5, 10) -> (2.5, -10)
  line L42 (2.5, -10) -> (7.5, -10)
  line L43 (7.5, -10) -> (7.5, 10)
  line L44 (7.5, 10) -> (2.5, -10) construction
  line L45 (2.5, 10) -> (7.5, -10) construction
  point P0 (-10, 0)
  point P1 (10, 0)
  point P2 (10, 0)
  point P3 (15, 0)
  point P4 (5, 0)
  dimension "d24" = 45
  dimension "d25" = 12.5
  dimension "d26" = 20
  dimension "d27" = 20
  dimension "d28" = 12.5
  dimension "d29" = 5
  dimension "d30" = 20
  dimension "d31" = 5
  dimension "d32" = 20
  constraint horizontal L0
  constraint perpendicular L0 L1
  constraint parallel L0 L2
  constraint parallel L1 L3
  constraint coincident L4 A0.centre
  constraint coincident L5 A0.centre
  constraint coincident A0.centre A2.centre
  constraint horizontal L6
  constraint vertical L7
  constraint horizontal L8
  constraint vertical L9
  constraint coincident L2 L7.end
  constraint horizontal L10
  constraint perpendicular L10 L11
  constraint parallel L10 L12
  constraint parallel L11 L13
  constraint coincident L14 P0
  constraint coincident L15 P0
  constraint horizontal L18
  constraint vertical L19
  constraint horizontal L20
  constraint vertical L21
  constraint coincident L2 L19.end
  constraint horizontal L22
  constraint perpendicular L22 L23
  constraint parallel L22 L24
  constraint parallel L23 L25
  constraint coincident L26 P2
  constraint coincident L27 P2
  constraint midpoint L19 P2
  constraint horizontal L28
  constraint perpendicular L28 L29
  constraint parallel L28 L30
  constraint parallel L29 L31
  constraint coincident L32 P2
  constraint coincident L33 P2
  constraint coincident P2 P1
  constraint horizontal L34
  constraint perpendicular L34 L35
  constraint parallel L34 L36
  constraint parallel L35 L37
  constraint coincident L38 P3
  constraint coincident L39 P3
  constraint midpoint L31 P3
  constraint horizontal L40
  constraint perpendicular L40 L41
  constraint parallel L40 L42
  constraint parallel L41 L43
  constraint coincident L44 P4
  constraint coincident L45 P4
  constraint midpoint L29 P4
  measures "d24" distance of L1.end L2.end
  measures "d25" distance of L0.end L6.end
  measures "d26" distance of L11.end L12.end
  measures "d27" distance of L10.end L11.end
  measures "d28" distance of L0.start L18.end
  measures "d29" distance of L35.end L36.end
  measures "d30" distance of L34.end L35.end
  measures "d31" distance of L41.end L42.end
  measures "d32" distance of L40.end L41.end
extrude "Extrude6" cut sketch "Sketch9" against normal blind 0.5 contours L22 L24 L28 L30 L31 L34 L35 L36 L37 | L22 L24 L28 L29 L30 L40 L41 L42 L43 | L7 L16 L17 | L7 L11 L16 L17 | L28 L30 L31 L35 | L28 L29 L30 L43

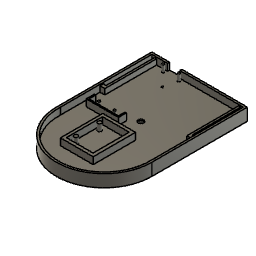
design "botton"
Autodesk Fusion 360 part; units mm, degrees
sketch "Sketch1" plane through (0, 0, 0) normal (0, 1, 0) x (1, 0, 0)
  line L0 (35, 35) -> (-35, 35)
  line L1 (-35, 35) -> (-35, -35)
  line L2 (-35, -35) -> (35, -35)
  line L3 (35, -35) -> (35, 35)
  line L4 (35, 35) -> (-35, -35) construction
  line L5 (-35, 35) -> (35, -35) construction
  circle A0 centre (0, -35) radius 35
  dimension "d1" = 70
  dimension "d2" = 70
  dimension "d3" = 70
  constraint horizontal L0
  constraint perpendicular L0 L1
  constraint parallel L0 L2
  constraint parallel L1 L3
  constraint coincident L4 origin
  constraint coincident L5 origin
  constraint midpoint L2 A0.centre
  measures "d1" distance of L1.end L2.end
  measures "d2" distance of L0.end L1.end
  measures "d3" diameter of A0
extrude "Extrude1" add sketch "Sketch1" along normal blind 4 makes body 1
sketch "Sketch2" plane through (0, 4, 0) normal (0, 1, 0) x (-1, 0, 0)
  line L0 (35, -35) -> (35, 35)
  arc A0 (35, 35) -> (-35, 35) centre (0, 35) ccw
  line L1 (-35, 35) -> (-35, -35)
  line L2 (-35, -35) -> (35, -35)
  line L3 (-35, -35) -> (35, -35)
  line L4 (35, -35) -> (35, 35)
  line L5 (35, 35) -> (-35, 35)
  line L6 (-35, 35) -> (-35, -35)
  line L7 (-35, -35) -> (35, 35) construction
  line L8 (35, -35) -> (-35, 35) construction
  circle A1 centre (0, 35) radius 35
  line L9 (-33.5, -33.5) -> (33.5, -33.5)
  line L10 (33.5, -33.5) -> (33.5, 33.5)
  line L11 (33.5, 33.5) -> (-33.5, 33.5)
  line L12 (-33.5, 33.5) -> (-33.5, -33.5)
  line L13 (-33.5, -33.5) -> (33.5, 33.5) construction
  line L14 (33.5, -33.5) -> (-33.5, 33.5) construction
  circle A2 centre (0, 35) radius 33.5
  dimension "d6" = 70
  dimension "d7" = 70
  dimension "d8" = 70
  dimension "d9" = 67
  dimension "d10" = 67
  dimension "d11" = 67
  constraint horizontal L3
  constraint perpendicular L3 L4
  constraint parallel L3 L5
  constraint parallel L4 L6
  constraint coincident L7 origin
  constraint coincident L8 origin
  constraint concentric A0 A1
  constraint horizontal L9
  constraint perpendicular L9 L10
  constraint parallel L9 L11
  constraint parallel L10 L12
  constraint coincident L13 origin
  constraint coincident L14 origin
  constraint concentric A1 A2
  measures "d6" distance of L0.end A0.end
  measures "d7" distance of L0.start L0.end
  measures "d8" diameter of A1
  measures "d9" distance of L10.end L11.end
  measures "d10" distance of L9.end L10.end
  measures "d11" diameter of A2
extrude "Extrude2" add sketch "Sketch2" along normal blind 5 contours L0 L1 L2 L3 L4 L6 A1 L9 L10 L12 | A0 L5 A1 A2 | L5 A1 L10 L11 A2 | L5 A1 L11 L12 A2 bodies 1